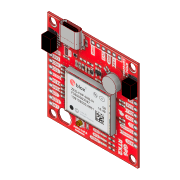
# Autodesk Inventor part: SparkFun GPS-RTK2 Board - ZED-F9P
Saved by Autodesk Inventor 2018 (Build 220112000, 112)
## iProperties
Created: 2019-02-06
Part Number: SparkFun GPS-RTK2 Board - ZED-F9P
Material: Generic
Document SubType Name: Modeling
Designer: Justin Hulbert
Density: 1 g/cm^3
Appearance: Smooth - Red
Author: Justin Hulbert
Autodesk Inventor part; units mm, degrees
ref_plane "YZ Plane" through (0, 0, 0) normal (1, 0, 0) x (0, 1, 0)
ref_plane "XZ Plane" through (0, 0, 0) normal (0, 1, 0) x (-1, 0, 0)
sketch "Sketch1" plane through (0, 0, 0) normal (0, 0, 1) x (1, 0, 0)
  line L0 (0, 0) -> (43.18, 0)
  line L1 (43.18, 0) -> (43.18, 43.18)
  line L2 (43.18, 43.18) -> (0, 43.18)
  line L3 (0, 43.18) -> (0, 0)
  dimension "d0" = 43.18
  dimension "d1" = 43.18
  constraints: 8 end point, 2 parallel, 1 horizontal, 1 perpendicular
  measures "d0" distance of L2.end L1.end
  measures "d1" distance of L1.end L0.end
extrude "Extrusion1" add sketch "Sketch1" along normal blind 0.762
sketch "Sketch2" plane through (0, 0, 0.762) normal (0, 0, 1) x (1, 0, 0)
  line L0 (0, 0) -> (43.18, 0) projected
  line L1 (43.18, 0) -> (43.18, 43.18) projected
  line L2 (43.18, 43.18) -> (0, 43.18) projected
  line L3 (0, 43.18) -> (0, 0) projected
  line L4 (2.54, 40.64) -> (40.64, 40.64)
  line L5 (40.64, 40.64) -> (40.64, 2.54)
  line L6 (40.64, 2.54) -> (2.54, 2.54)
  line L7 (2.54, 2.54) -> (2.54, 40.64)
  dimension "d4" = 2.54
  constraints: 8 end point, 4 coincident, 3 other
  measures "d4" distance between parallel lines of L2 L4
hole "Hole1" at (2.54, 40.64, 0.762) at (2.54, 2.54, 0.762) at (40.64, 2.54, 0.762) at (40.64, 40.64, 0.762) direction (0, 0, -1) diameter 3.3528 depth 25.4 tip angle 118
ref_plane "Work Plane1" through (0, 44.704, 0) normal (0, 1, 0) x (1, 0, 0)
sketch "Sketch3" plane through (0, 44.704, 0) normal (0, 1, 0) x (1, 0, 0)
  line L0 (43.18, -0.762) -> (0, -0.762) projected
  line L1 (9.4488, -0.762) -> (15.9512, -0.762)
  line L2 (17.2212, -2.032) -> (17.2212, -2.7432)
  line L3 (15.9512, -4.0132) -> (9.4488, -4.0132)
  line L4 (8.1788, -2.7432) -> (8.1788, -2.032)
  line L5 (0, 0) -> (0, -0.762) projected
  arc A0 (9.4488, -0.762) -> (8.1788, -2.032) centre (9.4488, -2.032) ccw
  arc A1 (17.2212, -2.032) -> (15.9512, -0.762) centre (15.9512, -2.032) ccw
  arc A2 (15.9512, -4.0132) -> (17.2212, -2.7432) centre (15.9512, -2.7432) ccw
  arc A3 (8.1788, -2.7432) -> (9.4488, -4.0132) centre (9.4488, -2.7432) ccw
  line L6 (0, -0.762) -> (43.18, -0.762) projected
  line L7 (12.827, -0.762) -> (12.827, 2.5763)
  line L8 (12.7, -4.0132) -> (12.7, -2.4751)
  point P0 (8.1788, -0.762)
  point P1 (17.2212, -4.0132)
  point P2 (17.2212, -0.762)
  point P3 (8.1788, -4.0132)
  dimension "d13" = 9.0424
  dimension "d14" = 3.2512
  dimension "d15" = 8.1788
  dimension "d16" = 1.27
  constraints: 12 end point, 10 point on line, 8 point on circle, 8 tangent, 4 centre point, 3 equal radius, 2 parallel, 2 vertical, 1 horizontal, 1 midpoint, 1 perpendicular
  measures "d13" distance of point (17.221, -4.013) point (8.179, -4.013)
  measures "d14" distance of point (17.221, -0.762) point (17.221, -4.013)
  measures "d15" distance between parallel lines of L4 L5
  measures "d16" radius of A0
extrude "Extrusion2" add sketch "Sketch3" against normal blind 7.366
sketch "Sketch4" plane through (0, 44.704, 0) normal (0, 1, 0) x (1, 0, 0)
  line L0 (9.4488, -0.762) -> (15.9512, -0.762) projected
  arc A0 (9.4488, -0.762) -> (8.1788, -2.032) centre (9.4488, -2.032) ccw projected
  line L1 (8.1788, -2.7432) -> (8.1788, -2.032) projected
  arc A1 (8.1788, -2.7432) -> (9.4488, -4.0132) centre (9.4488, -2.7432) ccw projected
  line L2 (15.9512, -4.0132) -> (9.4488, -4.0132) projected
  arc A2 (15.9512, -4.0132) -> (17.2212, -2.7432) centre (15.9512, -2.7432) ccw projected
  line L3 (17.2212, -2.032) -> (17.2212, -2.7432) projected
  arc A3 (17.2212, -2.032) -> (15.9512, -0.762) centre (15.9512, -2.032) ccw projected
  line L4 (9.4488, -2.032) -> (15.9512, -2.032)
  line L5 (15.9512, -2.032) -> (15.9512, -2.7432)
  line L6 (15.9512, -2.7432) -> (9.4488, -2.7432)
  line L7 (9.4488, -2.7432) -> (9.4488, -2.032)
  arc A4 (9.4488, -0.8459) -> (8.2627, -2.032) centre (9.4488, -2.032) ccw
  line L8 (9.4488, -0.8459) -> (15.9512, -0.8459)
  arc A5 (17.1373, -2.032) -> (15.9512, -0.8459) centre (15.9512, -2.032) ccw
  line L9 (17.1373, -2.032) -> (17.1373, -2.7432)
  arc A6 (15.9512, -3.9293) -> (17.1373, -2.7432) centre (15.9512, -2.7432) ccw
  line L10 (15.9512, -3.9293) -> (9.4488, -3.9293)
  arc A7 (8.2627, -2.7432) -> (9.4488, -3.9293) centre (9.4488, -2.7432) ccw
  line L11 (8.2627, -2.7432) -> (8.2627, -2.032)
  point P0 (0, 0)
  constraints: 16 end point, 8 point on circle, 4 centre point, 3 perpendicular, 1 horizontal, 7 other
extrude "Extrusion3" cut sketch "Sketch4" against normal blind 5.08 contours L8 A5 L9 A6 L10 A7 L11 A4
sketch "Sketch5" plane through (0, 0, 0.762) normal (0, 0, 1) x (1, 0, 0)
  line L0 (9.4488, 43.18) -> (9.4488, 37.338) projected
  line L1 (9.4488, 43.18) -> (0, 43.18) projected
  line L2 (0, 43.18) -> (0, 0) projected
  line L3 (0, 0) -> (43.18, 0) projected
  line L4 (43.18, 0) -> (43.18, 43.18) projected
  line L5 (43.18, 43.18) -> (15.9512, 43.18) projected
  line L6 (15.9512, 43.18) -> (15.9512, 37.338) projected
  line L7 (15.9512, 37.338) -> (9.4488, 37.338) projected
  circle A0 centre (40.64, 2.54) radius 1.6764 projected
  circle A1 centre (2.54, 40.64) radius 1.6764 projected
  circle A2 centre (2.54, 2.54) radius 1.6764 projected
  circle A3 centre (40.64, 40.64) radius 1.6764 projected
  line L8 (0, 0) -> (43.18, 0) projected
  line L9 (21.59, 0) -> (21.59, 11.5828)
  line L10 (0.254, 35.6558) -> (4.4958, 35.6558)
  line L11 (4.4958, 35.6558) -> (4.4958, 29.6868)
  line L12 (4.4958, 29.6868) -> (0.254, 29.6868)
  line L13 (0.254, 29.6868) -> (0.254, 35.6558)
  line L14 (42.926, 35.6558) -> (38.6842, 35.6558)
  line L15 (38.6842, 35.6558) -> (38.6842, 29.6868)
  line L16 (38.6842, 29.6868) -> (42.926, 29.6868)
  line L17 (42.926, 29.6868) -> (42.926, 35.6558)
  dimension "d21" = 4.2418
  dimension "d22" = 5.969
  dimension "d23" = 0.254
  constraints: 18 end point, 4 symmetric about line, 2 parallel, 1 horizontal, 1 midpoint, 1 perpendicular, 1 vertical
  measures "d21" distance of L11.end L12.end
  measures "d22" distance of L10.end L11.end
  measures "d23" distance between parallel lines of L2 L13
extrude "Extrusion4" add sketch "Sketch5" along normal blind 3.0734 contours L10 L11 L12 L13 | L17 L16 L15 L14
sketch "Sketch6" plane through (0, 0, 0.762) normal (0, 0, 1) x (1, 0, 0)
  circle A0 centre (8.128, 4.064) radius 3.1877
  line L0 (0, 43.18) -> (0, 0) projected
  line L1 (0, 0) -> (43.18, 0) projected
  line L2 (6.526, 1.3081) -> (9.73, 1.3081)
  line L3 (8.128, 7.2517) -> (14.0521, 7.2517)
  dimension "d26" = 6.3754
  dimension "d27" = 8.128
  dimension "d28" = 4.064
  dimension "d29" = 5.9436
  constraints: 4 end point, 3 point on circle, 2 horizontal, 1 centre point, 1 tangent
  measures "d26" diameter of A0
  measures "d27" distance from line of A0.centre L0
  measures "d28" distance from line of A0.centre L1
  measures "d29" distance between parallel lines of L2 L3
extrude "Extrusion5" cut sketch "Sketch6" against normal through all contours A0 L2 picked at (8.128, 3.2893)
sketch "Sketch7" plane through (0, 0, 0.762) normal (0, 0, 1) x (1, 0, 0)
  line L0 (10.7696, 26.289) -> (32.7406, 26.289)
  line L1 (32.7406, 26.289) -> (32.7406, 9.271)
  line L2 (32.7406, 9.271) -> (10.7696, 9.271)
  line L3 (10.7696, 9.271) -> (10.7696, 26.289)
  line L4 (0, 0) -> (43.18, 0) projected
  line L5 (0, 43.18) -> (0, 0) projected
  dimension "d32" = 21.971
  dimension "d33" = 17.018
  dimension "d34" = 9.271
  dimension "d35" = 10.7696
  constraints: 8 end point, 2 parallel, 1 horizontal, 1 perpendicular
  measures "d32" distance of L1.end L2.end
  measures "d33" distance of L0.end L1.end
  measures "d34" distance between parallel lines of L4 L2
  measures "d35" distance between parallel lines of L5 L3
extrude "Extrusion6" add sketch "Sketch7" along normal blind 2.5908
sketch "Sketch8" plane through (0, 0, 0.762) normal (0, 0, 1) x (1, 0, 0)
  circle A0 centre (32.004, 30.1752) radius 3.3782
  line L0 (43.18, 43.18) -> (15.9512, 43.18) projected
  line L1 (43.18, 0) -> (43.18, 43.18) projected
  point P0 (0, 0)
  dimension "d38" = 6.7564
  dimension "d39" = 13.0048
  dimension "d40" = 11.176
  constraints: 1 centre point
  measures "d38" diameter of A0
  measures "d39" distance from line of L0 A0.centre
  measures "d40" distance from line of L1 A0.centre
extrude "Extrusion7" add sketch "Sketch8" along normal blind 2.5908
sketch "Sketch9" plane through (0, 0, 0.762) normal (0, 0, 1) x (1, 0, 0)
  circle A0 centre (15.748, 5.334) radius 0.9906
  circle A1 centre (15.748, 5.334) radius 0.8567
  circle A2 centre (15.748, 5.334) radius 0.3208
  line L0 (0, 43.18) -> (0, 0) projected
  line L1 (0, 0) -> (43.18, 0) projected
  dimension "d43" = 1.9812
  dimension "d44" = 15.748
  dimension "d45" = 5.334
  constraints: 3 centre point, 2 coincident
  measures "d43" diameter of A0
  measures "d44" distance from line of L0 A0.centre
  measures "d45" distance from line of L1 A0.centre
extrude "Extrusion8" add sketch "Sketch9" along normal blind 1.27
sketch "Sketch10" plane through (9.4488, 44.704, 4.0132) normal (0, 0, 1) x (1, 0, 0)
  line L0 (-9.4517, -1.8915) -> (33.7316, -1.8915) construction
  line L1 (33.7316, -1.8915) -> (33.7316, -44.7034) construction
  line L2 (33.7316, -44.7034) -> (-9.4517, -44.7034) construction
  line L3 (-9.4517, -44.7034) -> (-9.4517, -1.8915) construction
  point P0 (-9.4488, -44.704)
  constraints: 2 other
decal "Decal1"
sketch "Sketch11" plane through (0, 0, 3.3528) normal (0, 0, 1) x (1, 0, 0)
  line L0 (0.004, 42.7411) -> (43.1873, 42.7411) construction
  line L1 (43.1873, 42.7411) -> (43.1873, -0.0708) construction
  line L2 (43.1873, -0.0708) -> (0.004, -0.0708) construction
  line L3 (0.004, -0.0708) -> (0.004, 42.7411) construction
  point P0 (0, 0)
  point P1 (-9.4488, -44.704)
  constraints: 2 other
decal "Decal2"
body "Solid1"
